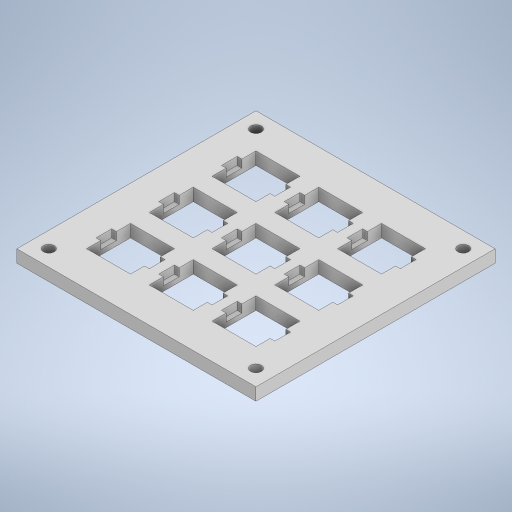
# Autodesk Inventor part: Keypad part 1
Saved by Autodesk Inventor 2023 (Build 270158000, 158)
## iProperties
Created: 2022-12-19
Part Number: Keypad part 1
Material: Generic
Document SubType Name: Modeling
Designer: appab
Density: 1 g/cm^3
Appearance: Default
Author: appab
Autodesk Inventor part; units mm, degrees
ref_plane "YZ Plane" through (0, 0, 0) normal (1, 0, 0) x (0, 1, 0)
ref_plane "XZ Plane" through (0, 0, 0) normal (0, 1, 0) x (-1, 0, 0)
ref_plane "XY Plane" through (0, 0, 0) normal (0, 0, 1) x (1, 0, 0)
sketch "Sketch1" plane through (0, 0, 0) normal (0, 1, 0) x (-1, 0, 0)
  line L0 (0, 0) -> (-14, 0)
  line L1 (-14, 0) -> (-14, -14)
  line L2 (-14, -14) -> (0, -14)
  line L3 (0, -14) -> (0, 0)
  line L4 (0, -20) -> (-14, -20)
  line L5 (0, -34) -> (0, -20)
  line L6 (-14, -34) -> (0, -34)
  line L7 (-14, -20) -> (-14, -34)
  line L8 (0, -40) -> (-14, -40)
  line L9 (0, -54) -> (0, -40)
  line L10 (-14, -54) -> (0, -54)
  line L11 (-14, -40) -> (-14, -54)
  line L12 (-20, 0) -> (-34, 0)
  line L13 (-20, -14) -> (-20, 0)
  line L14 (-34, -14) -> (-20, -14)
  line L15 (-34, 0) -> (-34, -14)
  line L16 (-20, -20) -> (-34, -20)
  line L17 (-20, -34) -> (-20, -20)
  line L18 (-34, -34) -> (-20, -34)
  line L19 (-34, -20) -> (-34, -34)
  line L20 (-20, -40) -> (-34, -40)
  line L21 (-20, -54) -> (-20, -40)
  line L22 (-34, -54) -> (-20, -54)
  line L23 (-34, -40) -> (-34, -54)
  line L24 (-40, 0) -> (-54, 0)
  line L25 (-40, -14) -> (-40, 0)
  line L26 (-54, -14) -> (-40, -14)
  line L27 (-54, 0) -> (-54, -14)
  line L28 (-40, -20) -> (-54, -20)
  line L29 (-40, -34) -> (-40, -20)
  line L30 (-54, -34) -> (-40, -34)
  line L31 (-54, -20) -> (-54, -34)
  line L32 (-40, -40) -> (-54, -40)
  line L33 (-40, -54) -> (-40, -40)
  line L34 (-54, -54) -> (-40, -54)
  line L35 (-54, -40) -> (-54, -54)
  line L36 (-59.4, -59.4) -> (-59.4, 5.4)
  line L37 (-59.4, 5.4) -> (5.4, 5.4)
  line L38 (5.4, 5.4) -> (5.4, -59.4)
  line L39 (5.4, -59.4) -> (-59.4, -59.4)
  line L40 (0, -20) -> (0, -14)
  line L41 (-14, 0) -> (-20, 0)
  dimension "d0" = 14
  dimension "d1" = 14
  dimension "d4" = 20
  dimension "d7" = 20
  dimension "d10" = 25.4
  constraints: 84 end point, 2 collinear, 2 horizontal, 2 parallel, 2 perpendicular, 1 vertical, 65 other
  measures "d0" distance of L2.end L1.end
  measures "d1" distance of L1.end L0.end
  measures "d4" distance of L0.start L4.start
  measures "d7" distance of L0.start L12.start
  measures "d10" distance between parallel lines of L19 L36
extrude "Extrusion1" add sketch "Sketch1" along normal blind 4
sketch "Sketch2" plane through (0, 0, 0) normal (0, -1, 0) x (1, 0, 0)
  line L0 (34, -20) -> (20, -20) construction
  line L1 (20, -20) -> (20, -34) construction
  line L2 (34, -20) -> (20, -34) construction
  line L3 (65.1, 11.1) -> (-11.1, 11.1)
  line L4 (-11.1, 11.1) -> (-11.1, -65.1)
  line L5 (-11.1, -65.1) -> (65.1, -65.1)
  line L6 (65.1, -65.1) -> (65.1, 11.1)
  line L7 (65.1, 11.1) -> (-11.1, -65.1) construction
  line L8 (-11.1, 11.1) -> (65.1, -65.1) construction
  line L9 (59.4, 5.4) -> (-5.4, 5.4)
  line L10 (-5.4, 5.4) -> (-5.4, -59.4)
  line L11 (-5.4, -59.4) -> (59.4, -59.4)
  line L12 (59.4, -59.4) -> (59.4, 5.4)
  line L13 (59.4, 5.4) -> (-5.4, -59.4) construction
  line L14 (-5.4, 5.4) -> (59.4, -59.4) construction
  point P0 (0, 0)
  point P1 (27, -27)
  dimension "d13" = 76.2
  constraints: 26 end point, 5 midpoint, 4 parallel, 2 horizontal, 2 perpendicular, 1 point on line
  measures "d13" distance of L5.end L4.end
extrude "Extrusion2" add sketch "Sketch2" against normal blind 4
sketch "Sketch3" plane through (0, 4, 0) normal (0, 1, 0) x (1, 0, 0)
  line L0 (54, 54) -> (54, 40) projected
  line L1 (54, 49.5) -> (55.5, 49.5)
  line L2 (55.5, 49.5) -> (55.5, 44.5)
  line L3 (55.5, 44.5) -> (54, 44.5)
  line L4 (54, 44.5) -> (54, 49.5)
  line L5 (40, 40) -> (40, 54) construction
  line L6 (40, 49.5) -> (38.5, 49.5)
  line L7 (38.5, 49.5) -> (38.5, 44.5)
  line L8 (38.5, 44.5) -> (40, 44.5)
  line L9 (40, 44.5) -> (40, 49.5)
  line L10 (54, 40) -> (40, 40) projected
  line L11 (54, 40) -> (40, 40)
  line L12 (54, 29.5) -> (55.5, 29.5)
  line L13 (55.5, 29.5) -> (55.5, 24.5)
  line L14 (54, 24.5) -> (54, 29.5)
  line L15 (55.5, 24.5) -> (54, 24.5)
  line L16 (40, 24.5) -> (40, 29.5)
  line L17 (40, 29.5) -> (38.5, 29.5)
  line L18 (38.5, 29.5) -> (38.5, 24.5)
  line L19 (38.5, 24.5) -> (40, 24.5)
  line L20 (54, 9.5) -> (55.5, 9.5)
  line L21 (55.5, 9.5) -> (55.5, 4.5)
  line L22 (54, 4.5) -> (54, 9.5)
  line L23 (55.5, 4.5) -> (54, 4.5)
  line L24 (40, 4.5) -> (40, 9.5)
  line L25 (40, 9.5) -> (38.5, 9.5)
  line L26 (38.5, 9.5) -> (38.5, 4.5)
  line L27 (38.5, 4.5) -> (40, 4.5)
  line L28 (34, 49.5) -> (35.5, 49.5)
  line L29 (35.5, 49.5) -> (35.5, 44.5)
  line L30 (34, 44.5) -> (34, 49.5)
  line L31 (35.5, 44.5) -> (34, 44.5)
  line L32 (20, 44.5) -> (20, 49.5)
  line L33 (20, 49.5) -> (18.5, 49.5)
  line L34 (18.5, 49.5) -> (18.5, 44.5)
  line L35 (18.5, 44.5) -> (20, 44.5)
  line L36 (34, 29.5) -> (35.5, 29.5)
  line L37 (35.5, 29.5) -> (35.5, 24.5)
  line L38 (34, 24.5) -> (34, 29.5)
  line L39 (35.5, 24.5) -> (34, 24.5)
  line L40 (20, 24.5) -> (20, 29.5)
  line L41 (20, 29.5) -> (18.5, 29.5)
  line L42 (18.5, 29.5) -> (18.5, 24.5)
  line L43 (18.5, 24.5) -> (20, 24.5)
  line L44 (34, 9.5) -> (35.5, 9.5)
  line L45 (35.5, 9.5) -> (35.5, 4.5)
  line L46 (34, 4.5) -> (34, 9.5)
  line L47 (35.5, 4.5) -> (34, 4.5)
  line L48 (20, 4.5) -> (20, 9.5)
  line L49 (20, 9.5) -> (18.5, 9.5)
  line L50 (18.5, 9.5) -> (18.5, 4.5)
  line L51 (18.5, 4.5) -> (20, 4.5)
  line L52 (14, 49.5) -> (15.5, 49.5)
  line L53 (15.5, 49.5) -> (15.5, 44.5)
  line L54 (14, 44.5) -> (14, 49.5)
  line L55 (15.5, 44.5) -> (14, 44.5)
  line L56 (0, 44.5) -> (0, 49.5)
  line L57 (0, 49.5) -> (-1.5, 49.5)
  line L58 (-1.5, 49.5) -> (-1.5, 44.5)
  line L59 (-1.5, 44.5) -> (0, 44.5)
  line L60 (14, 29.5) -> (15.5, 29.5)
  line L61 (15.5, 29.5) -> (15.5, 24.5)
  line L62 (14, 24.5) -> (14, 29.5)
  line L63 (15.5, 24.5) -> (14, 24.5)
  line L64 (0, 24.5) -> (0, 29.5)
  line L65 (0, 29.5) -> (-1.5, 29.5)
  line L66 (-1.5, 29.5) -> (-1.5, 24.5)
  line L67 (-1.5, 24.5) -> (0, 24.5)
  line L68 (14, 9.5) -> (15.5, 9.5)
  line L69 (15.5, 9.5) -> (15.5, 4.5)
  line L70 (14, 4.5) -> (14, 9.5)
  line L71 (15.5, 4.5) -> (14, 4.5)
  line L72 (0, 4.5) -> (0, 9.5)
  line L73 (0, 9.5) -> (-1.5, 9.5)
  line L74 (-1.5, 9.5) -> (-1.5, 4.5)
  line L75 (-1.5, 4.5) -> (0, 4.5)
  point P0 (0, 0)
  dimension "d16" = 1.5
  dimension "d17" = 5
  dimension "d18" = 1.5
  dimension "d19" = 5
  dimension "d22" = 20
  dimension "d25" = 20
  constraints: 146 end point, 4 horizontal, 4 parallel, 2 perpendicular, 2 point on line, 1 vertical, 128 other
  measures "d16" distance of L2.end L3.end
  measures "d17" distance of L1.end L2.end
  measures "d18" distance of L8.end L7.end
  measures "d19" distance of L7.end L6.end
  measures "d22" distance of L1.start L12.start
  measures "d25" distance of L1.start L28.start
extrude "Extrusion3" cut sketch "Sketch3" against normal blind 2.5
sketch "Sketch4" plane through (0, 4, 0) normal (0, 1, 0) x (1, 0, 0)
  line L0 (65.1, -11.1) -> (65.1, 65.1) projected
  line L1 (65.1, -11.1) -> (54.94, -11.1)
  line L2 (54.94, -11.1) -> (54.94, -0.94)
  line L3 (54.94, -0.94) -> (65.1, -0.94)
  line L4 (65.1, -0.94) -> (65.1, -11.1)
  circle A0 centre (60.02, -6.02) radius 1.7399
  circle A1 centre (60.02, 60.02) radius 1.7399
  circle A2 centre (-6.02, -6.02) radius 1.7399
  circle A3 centre (-6.02, 60.02) radius 1.7399
  point P0 (0, 0)
  dimension "d30" = 10.16
  dimension "d31" = 10.16
  dimension "d32" = 3.4798
  dimension "d35" = 66.04
  dimension "d38" = 66.04
  constraints: 8 end point, 4 centre point, 2 horizontal, 2 parallel, 1 perpendicular, 1 vertical, 6 other
  measures "d30" distance of L2.end L3.end
  measures "d31" distance of L1.end L2.end
  measures "d32" diameter of A0
  measures "d35" distance of A0.centre A1.centre
  measures "d38" distance of A0.centre A2.centre
extrude "Extrusion4" cut sketch "Sketch4" against normal blind 4 contours A0 | A1 | A2 | A3
body "Solid1"
